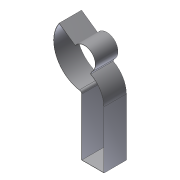
# Autodesk Inventor part: SketchProfile
Saved by Autodesk Inventor 2012 (Build 160160000, 160)
## iProperties
Created: 2012-01-20
Part Number: SketchProfile
Material: Default
Document SubType Name: Modeling
Designer: JesseK
Density: 1 g/cm^3
Mass: 1388.17 g
Surface Area: 11067.1 cm^2
Volume: 1388.17 cm^3
Author: JesseK
Autodesk Inventor part; units mm, degrees
ref_plane "YZ Plane" through (0, 0, 0) normal (1, 0, 0) x (0, 1, 0)
ref_plane "XZ Plane" through (0, 0, 0) normal (0, 1, 0) x (-1, 0, 0)
ref_plane "XY Plane" through (0, 0, 0) normal (0, 0, 1) x (1, 0, 0)
sketch "Sketch1" plane through (0, 0, 0) normal (0, 0, 1) x (1, 0, 0)
  circle A0 centre (330.2, 1028.7) radius 101.6
  arc A1 (101.3289, 1188.9573) -> (284.1769, 753.1166) centre (330.2, 1028.7) ccw
  circle A2 centre (285.75, 734.1316) radius 19.05
  line L0 (330.2, 1028.7) -> (431.8, 1028.7) construction
  line L1 (0, 1023.3941) -> (50.8, 1023.3941)
  line L2 (50.8, 1023.3941) -> (50.8, 972.5941)
  line L3 (50.8, 972.5941) -> (0, 972.5941)
  line L4 (0, 972.5941) -> (0, 1023.3941)
  line L5 (0, 0) -> (685.8, 0) construction
  line L6 (685.8, 1498.6) -> (0, 1498.6) construction
  line L7 (0, 1498.6) -> (0, 0) construction
  line L8 (304.8, 734.1316) -> (304.8, 213.868)
  line L9 (101.3289, 1188.9573) -> (318.1431, 1498.6) construction
  line L10 (101.3289, 1188.9573) -> (685.8, 1188.9573) construction
  arc A3 (508, 734.1316) -> (260.3446, 954.9248) centre (285.75, 734.1316) ccw
  line L11 (508, 734.1316) -> (508, 213.868)
  line L12 (685.8, 1188.9573) -> (685.8, 0) construction
  line L13 (685.8, 228.9727) -> (685.8, 178.1727)
  line L14 (101.3289, 1188.9573) -> (246.9742, 1086.9754)
  line L15 (304.8, 213.868) -> (508, 213.868)
  arc A4 (401.1312, 955.9585) -> (387.7592, 931.5884) centre (434.38, 921.8609) ccw
  dimension "d0" = 203.2
  dimension "d1" = 279.4
  dimension "d3" = 50.8
  dimension "d4" = 1498.6
  dimension "d5" = 685.8
  dimension "d6" = 38.1
  dimension "d9" = 55
  dimension "d10" = 1028.7
  dimension "d14" = 213.868
  dimension "d20" = 304.8
  dimension "d21" = 177.8
  constraints: 32 end point, 13 point on circle, 5 centre point, 5 horizontal, 5 tangent, 3 parallel, 3 perpendicular, 3 vertical, 2 coincident, 2 collinear, 1 point on line
  measures "d0" diameter of A0
  measures "d1" radius of A1
  measures "d3" distance of L3.end L1.start
  measures "d4" distance of L6.end L5.start
  measures "d5" distance of L5.start L5.end
  measures "d6" diameter of A2
  measures "d9" angle of L10 L9
  measures "d10" distance from line of L5 A0.centre
  measures "d14" distance between parallel lines of L15 L5
  measures "d20" distance between parallel lines of L7 L8
  measures "d21" distance between parallel lines of L12 L11
extrude "Extrusion1" add sketch "Sketch1" along normal blind 203.2 contours A0 A3 | A0 A3 L11 L15 L8 A2 A1 L14 | A4 A3 A0 | A3 A0
shell "Shell1" thickness 2.54 removed faces 2 at (372.5333, 560.7104, 0) at (440.2667, 387.2892, 203.2)
body "Solid1"
